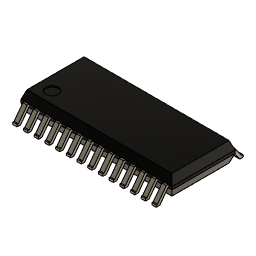
Adafruit 0.56in I2C 4 digit 7 segment LED (Autodesk Fusion 360 archive; units mm, degrees)
design "SOP28_300mil"
Autodesk Fusion 360 part; units mm, degrees
sketch "Sketch2" plane through (0, 0, 0) normal (1, 0, 0) x (0, 1, 0)
  line L0 (-3.7465, 0.3048) -> (3.7465, 0.3048)
  line L1 (3.7465, 0.3048) -> (3.7465, 2.6416)
  line L2 (3.7465, 2.6416) -> (-3.7465, 2.6416)
  line L3 (-3.7465, 2.6416) -> (-3.7465, 0.3048)
  line L4 (0, 2.6416) -> (0, 0.3048) construction
  line L5 (3.7465, 1.4732) -> (-3.7465, 1.4732) construction
  dimension "d3" = 7.493
  dimension "d4" = 2.3368
  dimension "d5" = 2.6416
  constraint horizontal L0
  constraint vertical L1
  constraint horizontal L2
  constraint vertical L3
  constraint midpoint L2 L4.start
  constraint midpoint L0 L4.end
  constraint midpoint L1 L5.start
  constraint midpoint L3 L5.end
  measures "d3" distance of L1.end L2.end
  measures "d4" distance of L0.start L2.end
  measures "d5" distance of origin L2
extrude "Extrude1" add sketch "Sketch2" along normal blind 8.9535 and the other way blind 8.9535 makes body 1
chamfer "Chamfer1" distance 0.9982 angle 20 4 edges at (0, -3.7465, 2.6416) (-8.9535, 0, 2.6416) (0, 3.7465, 2.6416) (8.9535, 0, 2.6416) measured on face at (-2.9845, -3.7465, 1.8627) measured on face at (-8.9535, 1.2488, 1.0837) measured on face at (2.9845, 3.7465, 1.8627) measured on face at (8.9535, 1.2488, 1.0837) on bodies 1
chamfer "Chamfer2" distance 1.0033 angle 20 3 edges at (8.9535, 0, 0.3048) (0, -3.7465, 0.3048) (-8.9535, 0, 0.3048) measured on face at (8.9535, -1.2488, 1.1972) measured on face at (2.9845, -3.7465, 0.751) measured on face at (-8.9535, -1.2488, 1.1972) on bodies 1
chamfer "Chamfer3" distance 0.3683 angle 70 1 edges at (0, 3.7465, 0.3048) measured on face at (-2.8628, -1.0054, 0.3048) on bodies 1
sketch "Sketch3" plane through (0, 0, 2.6416) normal (0, 0, 1) x (-1, 0, 0)
  line L0 (8.5902, 3.3832) -> (-8.5902, 3.3832)
  line L1 (-8.5902, 3.3832) -> (-8.5902, -3.3832)
  line L2 (-8.5902, -3.3832) -> (8.5902, -3.3832)
  line L3 (8.5902, -3.3832) -> (8.5902, 3.3832)
  circle A0 centre (7, 2) radius 0.75
  dimension "d16" = 1.5
  measures "d16" diameter of A0
extrude "Extrude2" cut sketch "Sketch3" against normal blind 0.15 contours A0 bodies 1
sketch "Sketch4" plane through (0, 0, 2.6416) normal (0, 0, 1) x (-1, 0, 0)
  circle A0 centre (7, 2) radius 0.75
  line L0 (8.5902, 3.3832) -> (-8.5902, 3.3832)
  line L1 (-8.5902, 3.3832) -> (-8.5902, -3.3832)
  line L2 (-8.5902, -3.3832) -> (8.5902, -3.3832)
  line L3 (8.5902, -3.3832) -> (8.5902, 3.3832)
sketch "Sketch5" plane through (0, 0, 0) normal (1, 0, 0) x (0, 1, 0)
  line L0 (0, 4) -> (0, -1.5) construction
  line L1 (-3.4562, 1.6434) -> (-3.9562, 1.6434)
  line L2 (-3.9562, 1.6434) -> (-5.0062, 0.2434)
  line L3 (-5.0062, 0.2434) -> (-5.1562, 0.2434)
  line L4 (-5.1562, 0.2434) -> (-5.1562, 0)
  line L5 (-5.1562, 0) -> (-4.7498, 0)
  line L6 (-4.7498, 0) -> (-3.7687, 1.3081)
  line L7 (-3.7687, 1.3081) -> (-3.4562, 1.3081)
  line L8 (-3.4562, 1.3081) -> (-3.4562, 1.6434)
  line L9 (-3.7465, 1.6434) -> (3.7465, 1.6434)
  line L10 (3.7434, 1.3081) -> (-3.7465, 1.3081)
  line L11 (4.7498, 0) -> (3.7687, 1.3081)
  line L12 (3.4562, 1.3081) -> (3.4562, 1.6434)
  line L13 (5.1562, 0.2434) -> (5.1562, 0)
  line L14 (5.1562, 0) -> (4.7498, 0)
  line L15 (3.9562, 1.6434) -> (5.0062, 0.2434)
  line L16 (5.0062, 0.2434) -> (5.1562, 0.2434)
  line L17 (3.4562, 1.6434) -> (3.9562, 1.6434)
  line L18 (3.7687, 1.3081) -> (3.4562, 1.3081)
  point P0 (3.7465, 1.6434)
  point P1 (3.7465, 1.3081)
  dimension "d19" = 5.1562
  dimension "d20" = 0.4064
  constraint vertical L0
  constraint horizontal L1
  constraint parallel L1 L3
  constraint perpendicular L3 L4
  constraint perpendicular L4 L5
  constraint parallel L3 L7
  constraint perpendicular L7 L8
  constraint collinear L1 L9
  constraint collinear L7 L10
  constraint coincident origin L5
  constraint symmetric L0 L1.start L12.end
  constraint symmetric L0 L1.end L15.start
  constraint symmetric L0 L2.end L15.end
  constraint symmetric L0 L3.end L13.start
  constraint symmetric L0 L4.end L13.end
  constraint symmetric L0 L5.end L11.start
  constraint symmetric L0 L6.end L11.end
  constraint symmetric L0 L7.end L12.start
  constraint symmetric L0 L9.start P0
  constraint symmetric L0 L10.end P1
  measures "d19" distance of origin L4.end
  measures "d20" distance of L4.end L5.end
extrude "Extrude3" add sketch "Sketch5" along normal blind 0.508 separate body contours L1 L2 L3 L4 L5 L6 L7 L8 L9 L10 makes body 2
extrude "Extrude4" add sketch "Sketch5" along normal blind 0.508 separate body contours L9 L10 L11 L12 L13 L14 L15 L16 L17 L18 makes body 3
move_body "Move1" bodies 3 2 to x (1, 0, 0) y (0, 1, 0) z (0, 0, 1) at (-0.254, 0, 0)
move_body "Move2" bodies 3 2 to x (1, 0, 0) y (0, 1, 0) z (0, 0, 1) at (-0.635, 0, 0)
move_body "Move3" bodies 2 3 to x (1, 0, 0) y (0, 1, 0) z (0, 0, 1) at (-8.89, 0, 0)
move_body "Move4" bodies 3 2 to x (1, 0, 0) y (0, 1, 0) z (0, 0, 1) at (1.27, 0, 0)
pattern_linear "R-Pattern1" count 14 spacing 1.27 along (1, 0, 0) of bodies 2 3 makes body 4 at (-7.0697, -4.3062, 1.1767) makes body 5 at (-5.7997, -4.3062, 1.1767) makes body 6 at (-4.5297, -4.3062, 1.1767) makes body 7 at (-3.2597, -4.3062, 1.1767) makes body 8 at (-1.9897, -4.3062, 1.1767) makes body 9 at (-0.7197, -4.3062, 1.1767) makes body 10 at (0.5503, -4.3062, 1.1767) makes body 11 at (1.8203, -4.3062, 1.1767) makes body 12 at (3.0903, -4.3062, 1.1767) makes body 13 at (4.3603, -4.3062, 1.1767) makes body 14 at (5.6303, -4.3062, 1.1767) makes body 15 at (6.9003, -4.3062, 1.1767) makes body 16 at (8.1703, -4.3062, 1.1767) makes body 17 at (-7.0697, 4.3062, 1.1767) makes body 18 at (-5.7997, 4.3062, 1.1767) makes body 19 at (-4.5297, 4.3062, 1.1767) makes body 20 at (-3.2597, 4.3062, 1.1767) makes body 21 at (-1.9897, 4.3062, 1.1767) makes body 22 at (-0.7197, 4.3062, 1.1767) makes body 23 at (0.5503, 4.3062, 1.1767) makes body 24 at (1.8203, 4.3062, 1.1767) makes body 25 at (3.0903, 4.3062, 1.1767) makes body 26 at (4.3603, 4.3062, 1.1767) makes body 27 at (5.6303, 4.3062, 1.1767) makes body 28 at (6.9003, 4.3062, 1.1767) makes body 29 at (8.1703, 4.3062, 1.1767)
named bodies: "Pin1", "Pin28", "Pin2", "Pin3", "Pin4", "Pin5", "Pin6", "Pin7", "Pin8", "Pin9", "Pin10", "Pin11", "Pin12", "Pin13", "Pin14", "Pin27", "Pin26", "Pin25", "Pin24", "Pin23", "Pin22", "Pin21", "Pin20", "Pin19", "Pin18", "Pin17", "Pin16", "Pin15"
